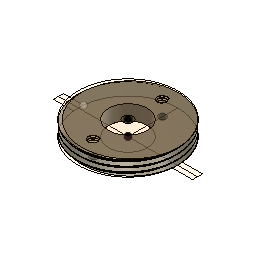
laser filter support mini v3 (Autodesk Fusion 360 design; units mm, degrees)
Autodesk Fusion 360 part; units mm, degrees
note: some values were not read from the file. Chosen so that the rebuilt part matches the saved one: where a thread starts. Set by a fixed rule: which face or edge a step refers to.
sketch "Sketch1" plane through (0, 0, 0) normal (0, 1, 0) x (1, 0, 0)
  circle A0 centre (0, 0) radius 10
  circle A1 centre (0, 0) radius 3.875
  line L0 (0, 0) -> (10, 0)
  line L1 (0, 0) -> (0, 3.875)
  line L2 (10, 0) -> (14, 0)
  line L3 (0, 0) -> (-10, 0)
  line L4 (-10, 0) -> (-14, 0)
  line L5 (14, 0) -> (14, 1)
  line L6 (14, 1) -> (14, -1)
  line L7 (14, -1) -> (9.9499, -1)
  line L8 (14, 1) -> (9.9499, 1)
  line L9 (-14, 0) -> (-14, 1)
  line L10 (-14, 1) -> (-14, -1)
  line L11 (-14, -1) -> (-9.9499, -1)
  line L12 (-14, 1) -> (-9.9499, 1)
  line L13 (0, 3.875) -> (0, 10)
  circle A2 centre (0, 6.9375) radius 0.75
  circle A3 centre (0, -6.9375) radius 0.75
  dimension "d1" = 20
  dimension "d2" = 7.75
  dimension "d3" = 4
  dimension "d4" = 4
  dimension "d5" = 1
  dimension "d6" = 2
  dimension "d7" = 1
  dimension "d8" = 2
  dimension "d9" = 1.5
  constraint coincident A0.centre A1.centre
  constraint coincident A0 L0.end
  constraint horizontal L0
  constraint coincident A1 L1.end
  constraint perpendicular L0 L1
  constraint parallel L0 L2
  constraint coincident A0 L3.end
  constraint perpendicular L1 L3
  constraint perpendicular L1 L4
  constraint perpendicular L2 L5
  constraint perpendicular L2 L6
  constraint coincident A0 L7.end
  constraint perpendicular L5 L7
  constraint coincident A0 L8.end
  constraint perpendicular L5 L8
  constraint perpendicular L4 L9
  constraint parallel L9 L10
  constraint coincident A0 L11.end
  constraint perpendicular L10 L11
  constraint perpendicular L10 L12
  constraint coincident A0 L13.end
  constraint parallel L1 L13
  constraint midpoint L13 A2.centre
  constraint symmetric L0 A2 A3
  measures "d1" diameter of A0
  measures "d2" diameter of A1
  measures "d3" distance of L0.end L2.end
  measures "d4" distance of L3.end L4.end
  measures "d5" distance of L2.end L5.end
  measures "d6" distance of L5.end L6.end
  measures "d7" distance of L4.end L9.end
  measures "d8" distance of L9.end L10.end
  measures "d9" diameter of A2
extrude "Extrude3" add sketch "Sketch1" along normal blind 3 contours A0 A1 L0 L13 A2 | A0 A1 L0 L3 | A0 A1 L3 L13 A2
thread "Thread3" "ISO Metric profile 20.0 M20x1 6g" major diameter 19.884 minor diameter 18.7405 pitch 1 angle 60 modelled right hand crest width 0.125 on face at (9.9901, 2, 0.445) crest through (9.942, -0.0625, 0)
thread "Thread4" "ISO Metric profile 2.0 M2x0.4 6H" major diameter 2.074 minor diameter 1.623 pitch 0.4 angle 60 modelled right hand crest width 0.05 on face at (0.7491, 2, 6.9749) crest through (0.8115, -0.225, 6.9375) on face at (-0.0374, 2, -6.1884) crest through (0.8115, -0.225, -6.9375)
sketch "Sketch3" plane through (0, 3, 0) normal (0, 1, 0) x (-1, 0, 0)
  spline S0 degree 3 poles (-7.0301, -7.0301) (-6.0949, -7.9147) (-4.9968, -8.6093) (-2.6081, -9.531) (-1.3425, -9.7542) (1.1894, -9.7006) (2.4312, -9.4296) (4.7275, -8.4299) (5.7619, -7.7157) (7.2001, -6.2349) (7.6925, -5.576) (8.4917, -4.153) (8.7966, -3.3957) (8.9998, -2.6086) knots 0 0 0 0 0.386194 0.386194 0.768284 0.768284 1.14627 1.14627 1.52015 1.52015 1.766131 1.766131 2.010278 2.010278 2.010278 2.010278
  arc A0 (8.9998, -2.6086) -> (4.5193, 8.2084) centre (0, 0) ccw
  spline S1 degree 3 poles (4.5193, 8.2084) (3.4628, 8.8313) (2.2942, 9.2406) (-0.1478, 9.5929) (-1.3983, 9.5272) (-3.8183, 8.9193) (-4.9631, 8.3777) (-6.9935, 6.8799) (-7.8565, 5.9339) (-8.9565, 4.123) (-9.3013, 3.3421) (-9.784, 1.7053) (-9.9183, 0.856) (-9.942, 0) knots 0 0 0 0 0.367945 0.367945 0.739991 0.739991 1.116138 1.116138 1.496385 1.496385 1.751172 1.751172 2.007788 2.007788 2.007788 2.007788
  arc A1 (-9.942, 0) -> (-7.0301, -7.0301) centre (0, 0) ccw
  spline S2 degree 3 poles (-0.8115, 6.9375) (-0.826, 7.0439) (-0.819, 7.1521) (-0.7636, 7.3654) (-0.7137, 7.4679) (-0.5749, 7.6531) (-0.4856, 7.7328) (-0.2774, 7.8572) (-0.1593, 7.8989) (0.0479, 7.9301) (0.1337, 7.9317) (0.306, 7.9127) (0.3916, 7.8917) (0.4736, 7.86) knots 0 0 0 0 0.032207 0.032207 0.066041 0.066041 0.101501 0.101501 0.138586 0.138586 0.164112 0.164112 0.190345 0.190345 0.190345 0.190345
  arc A2 (0.9872, 6.62) -> (0.4736, 7.86) centre (0, 6.9375) ccw
  spline S3 degree 3 poles (0.9872, 6.62) (0.9339, 6.4997) (0.858, 6.3907) (0.672, 6.2124) (0.5652, 6.1434) (0.3357, 6.0532) (0.2162, 6.031) (-0.0192, 6.0346) (-0.1328, 6.0582) (-0.3053, 6.1322) (-0.3683, 6.1692) (-0.4813, 6.2574) (-0.5312, 6.3076) (-0.5738, 6.3637) knots 0 0 0 0 0.039492 0.039492 0.077352 0.077352 0.11358 0.11358 0.148176 0.148176 0.170108 0.170108 0.191341 0.191341 0.191341 0.191341
  arc A3 (-0.8115, 6.9375) -> (-0.5738, 6.3637) centre (0, 6.9375) ccw
  spline S4 degree 3 poles (-0.8115, -6.9375) (-0.826, -6.8311) (-0.819, -6.7229) (-0.7636, -6.5096) (-0.7137, -6.4071) (-0.5749, -6.2219) (-0.4856, -6.1422) (-0.2774, -6.0178) (-0.1593, -5.9761) (0.0479, -5.9449) (0.1337, -5.9433) (0.306, -5.9623) (0.3916, -5.9833) (0.4736, -6.015) knots 0 0 0 0 0.032207 0.032207 0.066041 0.066041 0.101501 0.101501 0.138586 0.138586 0.164112 0.164112 0.190345 0.190345 0.190345 0.190345
  arc A4 (0.9872, -7.255) -> (0.4736, -6.015) centre (0, -6.9375) ccw
  spline S5 degree 3 poles (0.9872, -7.255) (0.9339, -7.3753) (0.858, -7.4843) (0.672, -7.6626) (0.5652, -7.7316) (0.3357, -7.8218) (0.2162, -7.844) (-0.0192, -7.8404) (-0.1328, -7.8168) (-0.3053, -7.7428) (-0.3683, -7.7058) (-0.4813, -7.6176) (-0.5312, -7.5674) (-0.5738, -7.5113) knots 0 0 0 0 0.039492 0.039492 0.077352 0.077352 0.11358 0.11358 0.148176 0.148176 0.170108 0.170108 0.191341 0.191341 0.191341 0.191341
  arc A5 (-0.8115, -6.9375) -> (-0.5738, -7.5113) centre (0, -6.9375) ccw
  circle A6 centre (0, 0) radius 3.875
  circle A7 centre (0, 0) radius 10
  circle A8 centre (0, 0) radius 1
  dimension "d18" = 20
  dimension "d19" = 2
  constraint concentric A0 A7
  constraint concentric A0 A8
  measures "d18" diameter of A7
  measures "d19" diameter of A8
extrude "Extrude1" [rolled back] along distance 6 taper angle 0
thread "Thread1" [rolled back]
extrude "Extrude2" [rolled back] along distance 4.25 taper angle 0
thread "Thread2" [rolled back] thread offset 0 thread length 4.25
